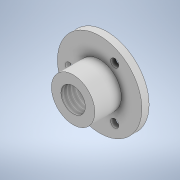
# Autodesk Inventor part: 製図規定課題2
Saved by Autodesk Inventor 2021 (Build 250183000, 183)
## iProperties
Created: 2021-10-03
Part Number: 製図規定課題2
Material: 一般
Document SubType Name: Modeling
Designer: ryusei
Density: 1 g/cm^3
Appearance: 既定
Author: ryusei
Autodesk Inventor part; units mm, degrees
ref_plane "YZ Plane" through (0, 0, 0) normal (1, 0, 0) x (0, 1, 0)
ref_plane "XZ Plane" through (0, 0, 0) normal (0, 1, 0) x (-1, 0, 0)
ref_plane "XY Plane" through (0, 0, 0) normal (0, 0, 1) x (1, 0, 0)
sketch "スケッチ1" plane through (0, 0, 0) normal (0, 0, 1) x (1, 0, 0)
  circle A0 centre (0, 0) radius 17.5
  dimension "d0" = 35
  constraints: 1 centre point, 1 coincident
  measures "d0" diameter of A0
extrude "押し出し1" add sketch "スケッチ1" along normal blind 3
sketch "スケッチ2" plane through (0, 0, 3) normal (0, 0, 1) x (1, 0, 0)
  circle A0 centre (0, 0) radius 9
  dimension "d3" = 18
  constraints: 1 centre point, 1 coincident
  measures "d3" diameter of A0
extrude "押し出し2" add sketch "スケッチ2" along normal blind 11
sketch "スケッチ3" plane through (0, 0, 14) normal (0, 0, 1) x (1, 0, 0)
  point P0 (0, 0)
  point P1 (0, 0)
  constraints: 1 coincident
hole "穴1" at (0, 0, 14) direction (0, 0, -1) diameter 10.106 end through all thread size "M12x1.75" class "6H" standard "ISO Metric profile"
sketch "スケッチ5" plane through (0, 0, 0) normal (0, 0, -1) x (-1, 0, 0)
  circle A0 centre (0, 0) radius 7
  dimension "d25" = 14
  constraints: 1 centre point, 1 coincident
  measures "d25" diameter of A0
extrude "押し出し3" cut sketch "スケッチ5" against normal blind 1
sketch "スケッチ6" plane through (0, 0, 0) normal (0, 0, -1) x (-1, 0, 0)
  point P0 (0, 0)
  point P1 (12.5, 0)
  point P2 (0, 0)
  point P3 (-6.25, 10.8253)
  point P4 (0, 0)
  point P5 (-6.25, -10.8253)
  dimension "d28" = 12.5
  dimension "d31" = 360
  constraints: 2 coincident, 5 other
  measures "d28" distance of point (0, 0) point (12.5, 0)
hole "穴3" at (-12.5, 0, 0) at (6.25, 10.8253, 0) at (6.25, -10.8253, 0) direction (0, 0, 1) diameter 3.4 end through all
sketch "スケッチ7" plane through (0, 0, 0) normal (0, 0, -1) x (-1, 0, 0)
  circle A0 centre (12.5, 0) radius 1.7 projected
  circle A1 centre (12.5, 0) radius 3
  circle A2 centre (-6.25, 10.8253) radius 3
  circle A3 centre (-6.25, -10.8253) radius 3
  point P0 (0, 0)
  dimension "d40" = 6
  dimension "d43" = 360
  constraints: 3 centre point, 1 coincident, 7 other
  measures "d40" diameter of A1
extrude "押し出し4" cut sketch "スケッチ7" against normal blind 1 contours A0 | A1 | A2 | A3
